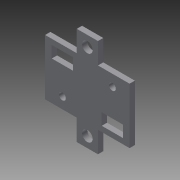
# Autodesk Inventor part: hook mount plate
Saved by Autodesk Inventor 2013 (Build 170138000, 138)
## iProperties
Created: 2013-01-26
Part Number: hook mount plate
Material: Generic
Document SubType Name: Modeling
Designer: Arpan
Density: 1 g/cm^3
Author: Arpan
Autodesk Inventor part; units mm, degrees
ref_plane "YZ Plane" through (0, 0, 0) normal (1, 0, 0) x (0, 1, 0)
ref_plane "XZ Plane" through (0, 0, 0) normal (0, 1, 0) x (-1, 0, 0)
ref_plane "XY Plane" through (0, 0, 0) normal (0, 0, 1) x (1, 0, 0)
sketch "Sketch1" plane through (0, 0, 0) normal (0, 0, 1) x (1, 0, 0)
  line L0 (76, 0) -> (0, 0)
  line L1 (76, -67) -> (0, -67)
  circle A0 centre (68, -13.5) radius 4.15
  circle A1 centre (8, -53.5) radius 4.15
  line L2 (68, -46.515) -> (55.3, -46.515)
  line L3 (55.3, -46.515) -> (55.3, -60.485)
  line L4 (55.3, -60.485) -> (80.7, -60.485)
  line L5 (80.7, -60.485) -> (80.7, -46.515)
  line L6 (80.7, -46.515) -> (68, -46.515)
  line L7 (76, 0) -> (88.7, 0)
  line L8 (88.7, 0) -> (88.7, -67)
  line L9 (88.7, -67) -> (76, -67)
  line L10 (0, 0) -> (-12.7, 0)
  line L11 (-12.7, 0) -> (-12.7, -67)
  line L12 (-12.7, -67) -> (0, -67)
  line L13 (-12.7, 0) -> (-12.7, -6.5024)
  line L14 (-12.7, -6.5024) -> (-4.699, -6.5024)
  line L15 (-4.699, -6.5024) -> (-4.699, -20.4724)
  line L16 (-4.699, -20.4724) -> (20.701, -20.4724)
  line L17 (20.701, -20.4724) -> (20.701, -6.5024)
  line L18 (20.701, -6.5024) -> (-4.699, -6.5024)
  line L19 (38, 25.4) -> (25.3, 25.4)
  line L20 (38, 25.4) -> (50.7, 25.4)
  line L21 (50.7, 25.4) -> (50.7, 0)
  line L22 (25.3, 25.4) -> (25.3, 0)
  line L23 (38, -67) -> (25.3, -67)
  line L24 (25.3, -67) -> (25.3, -92.4)
  line L25 (25.3, -92.4) -> (50.7, -92.4)
  line L26 (50.7, -92.4) -> (50.7, -67)
  line L27 (38, 0) -> (38, 12.7)
  circle A2 centre (38, 12.7) radius 6.35
  line L28 (38, -67) -> (38, -79.7)
  circle A3 centre (38, -79.7) radius 6.35
  point P0 (38, -33.5)
  dimension "d0" = 13.5
  dimension "d2" = 8.3
  dimension "d3" = 67
  dimension "d5" = 0
  dimension "d7" = 13.5
  dimension "d9" = 33.5
  dimension "d11" = 53.5
  dimension "d15" = 12.7
  dimension "d16" = 25.4
  dimension "d17" = 12.7
  dimension "d18" = 13.97
  dimension "d19" = 8
  dimension "d20" = 12.7
  dimension "d21" = 6.515
  dimension "d22" = 6.5024
  dimension "d23" = 8.001
  dimension "d24" = 13.97
  dimension "d26" = 25.4
  dimension "d27" = 67.999
  dimension "d28" = 88.7
  dimension "d29" = 12.7
  dimension "d30" = 20.7
  dimension "d31" = 50.7
  dimension "d32" = 80.7
  dimension "d33" = 88.7
  dimension "d37" = 12.7
  dimension "d38" = 12.7
  dimension "d39" = 25.4
  dimension "d40" = 25.4
  dimension "d41" = 12.7
  dimension "d42" = 12.7
  dimension "d43" = 12.7
  dimension "d44" = 12.7
  constraints: 58 end point, 10 perpendicular, 9 parallel, 6 point on line, 4 centre point, 3 collinear, 2 coincident, 2 midpoint, 1 equal radius, 1 horizontal
  measures "d0" distance from line of L0 A0.centre
  measures "d2" diameter of A0
  measures "d3" distance between parallel lines of L0 L1
  measures "d5" distance from line of point (0, 0) L0
  measures "d7" distance from line of A0.centre L0
  measures "d9" distance from line of point (38, -33.5) L0
  measures "d11" distance from line of A1.centre L0
  measures "d15" distance of L2.start L2.end
  measures "d16" distance of L3.end L4.end
  measures "d17" distance of L0.start L7.end
  measures "d18" distance of L2.end L3.end
  measures "d19" distance between parallel lines of L8 L5
  measures "d20" distance of L0.end L10.end
  measures "d21" distance between parallel lines of L4 L1
  measures "d22" distance of L10.end L13.end
  measures "d23" distance of L13.end L14.end
  measures "d24" distance of L14.end L15.end
  measures "d26" distance of L15.end L16.end
  measures "d27" distance between parallel lines of L8 L17
  measures "d28" distance from line of point (0, 0) L8
  measures "d29" distance from line of L1.start L8
  measures "d30" distance from line of A0.centre L8
  measures "d31" distance from line of point (38, -33.5) L8
  measures "d32" distance from line of A1.centre L8
  measures "d33" distance from line of L1.end L8
  measures "d37" distance of L19.start L19.end
  measures "d38" distance of L19.start L20.end
  measures "d39" distance of L19.end L22.end
  measures "d40" distance of L23.end L24.end
  measures "d41" distance of L27.start L27.end
  measures "d42" diameter of A2
  measures "d43" distance of L23.start L28.end
  measures "d44" diameter of A3
extrude "Extrusion2" add sketch "Sketch1" along normal blind 6.35
body "Solid2"
